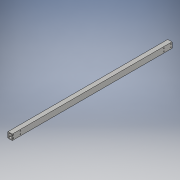
# Autodesk Inventor part: 前後機構_角柱1
Saved by Autodesk Inventor 2019.4 (Build 234330000, 330)
## iProperties
Created: 2021-12-05
Part Number: 前後機構_角柱1
Material: アルミニウム 6061
Document SubType Name: Modeling
Designer: 堀川皓史
Density: 2.7 g/cm^3
Appearance: アルミニウム - フラット
Author: 堀川皓史
Autodesk Inventor part; units mm, degrees
ref_plane "YZ Plane" through (0, 0, 0) normal (1, 0, 0) x (0, 1, 0)
ref_plane "XZ Plane" through (0, 0, 0) normal (0, 1, 0) x (-1, 0, 0)
ref_plane "XY Plane" through (0, 0, 0) normal (0, 0, 1) x (1, 0, 0)
sketch "スケッチ1" plane through (0, 0, 0) normal (0, 0, 1) x (1, 0, 0)
  line L0 (7.5, 10) -> (-7.5, 10)
  line L1 (-7.5, 10) -> (-7.5, -10)
  line L2 (-7.5, -10) -> (7.5, -10)
  line L3 (7.5, -10) -> (7.5, 10)
  line L4 (7.5, 10) -> (-7.5, -10) construction
  line L5 (-7.5, 10) -> (7.5, -10) construction
  line L6 (-5.5, 8) -> (5.5, 8)
  line L7 (5.5, 8) -> (5.5, -8)
  line L8 (5.5, -8) -> (-5.5, -8)
  line L9 (-5.5, -8) -> (-5.5, 8)
  point P0 (0, 0)
  dimension "d0" = 15
  dimension "d1" = 20
  dimension "d2" = 2
  constraints: 20 end point, 4 parallel, 2 midpoint, 2 perpendicular, 1 horizontal, 3 other
  measures "d0" distance of L2.end L1.end
  measures "d1" distance of L1.end L0.end
  measures "d2" distance between parallel lines of L0 L6
extrude "押し出し1" add sketch "スケッチ1" along normal blind 566
sketch "スケッチ2" plane through (7.5, -10, 0) normal (1, 0, 0) x (0, 0, -1)
  circle A0 centre (-4, 15) radius 1.6
  circle A1 centre (-4, 5) radius 1.6
  circle A2 centre (-29, 15) radius 1.6
  circle A3 centre (-29, 5) radius 1.6
  circle A4 centre (-537, 15) radius 1.6
  circle A5 centre (-537, 5) radius 1.6
  circle A6 centre (-562, 15) radius 1.6
  circle A7 centre (-562, 5) radius 1.6
  line L0 (-566, 0) -> (-566, 20) projected
  line L1 (0, 20) -> (-566, 20) projected
  point P0 (0, 10)
  dimension "d5" = 3.2
  dimension "d6" = 3.2
  dimension "d7" = 3.2
  dimension "d8" = 3.2
  dimension "d9" = 10
  dimension "d10" = 25
  dimension "d11" = 4
  dimension "d12" = 5
  dimension "d13" = 3.2
  dimension "d14" = 3.2
  dimension "d15" = 3.2
  dimension "d16" = 3.2
  dimension "d17" = 10
  dimension "d18" = 25
  dimension "d19" = 4
  dimension "d20" = 5
  constraints: 8 centre point, 4 horizontal alignment, 4 vertical alignment
  measures "d5" diameter of A0
  measures "d6" diameter of A1
  measures "d7" diameter of A2
  measures "d8" diameter of A3
  measures "d9" distance of A1.centre A0.centre
  measures "d10" distance of A0.centre A2.centre
  measures "d11" horizontal distance of point (0, 10) A1.centre
  measures "d12" vertical distance of point (0, 10) A1.centre
  measures "d13" diameter of A4
  measures "d14" diameter of A5
  measures "d15" diameter of A6
  measures "d16" diameter of A7
  measures "d17" distance of A5.centre A4.centre
  measures "d18" distance of A4.centre A6.centre
  measures "d19" distance from line of L0 A7.centre
  measures "d20" distance from line of L1 A6.centre
extrude "押し出し2" cut sketch "スケッチ2" against normal through all
